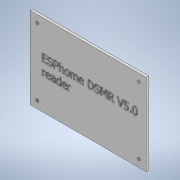
# Autodesk Inventor part: esp dsrm cover
Saved by Autodesk Inventor 2022.2 (Build 262287030, 287C)
## iProperties
Created: 2023-01-13
Part Number: esp dsrm cover
Material: Generic
Document SubType Name: Modeling
Designer: Ritchie
Density: 1 g/cm^3
Appearance: Default
Author: Ritchie
## iProperties of the stored document esp dsrm cover_3DPrint.ipt
Created: 2023-01-13
Part Number: esp dsrm cover_3DPrint
Material: Generic
Document SubType Name: Modeling
Designer: Ritchie
Density: 1 g/cm^3
Appearance: Default
Author: Ritchie
Autodesk Inventor part; units mm, degrees
ref_plane "YZ Plane" through (0, 0, 0) normal (1, 0, 0) x (0, 1, 0)
ref_plane "XZ Plane" through (0, 0, 0) normal (0, 1, 0) x (-1, 0, 0)
ref_plane "XY Plane" through (0, 0, 0) normal (0, 0, 1) x (1, 0, 0)
derived "esp_housing_dsrm.ipt"
sketch "Sketch15" plane through (0, 0, 33) normal (0, 0, 1) x (1, 0, 0)
  circle A0 centre (-9, 1) radius 1
  circle A1 centre (74.024, 55.742) radius 1
  circle A2 centre (-9, 55.742) radius 1
  arc A3 (77.024, 1) -> (74.024, -2) centre (74.024, 1) ccw
  line L0 (77.024, 1) -> (77.024, 55.742)
  arc A4 (74.024, 58.742) -> (77.024, 55.742) centre (74.024, 55.742) ccw
  line L1 (74.024, 58.742) -> (-9, 58.742)
  arc A5 (-12, 55.742) -> (-9, 58.742) centre (-9, 55.742) ccw
  line L2 (-12, 55.742) -> (-12, 1)
  arc A6 (-9, -2) -> (-12, 1) centre (-9, 1) ccw
  line L3 (-9, -2) -> (74.024, -2)
  circle A7 centre (74.024, 1) radius 1
  line L4 (-14, -4) -> (79.024, -4)
  line L5 (79.024, -4) -> (79.024, 60.742)
  line L6 (79.024, 60.742) -> (-14, 60.742)
  line L7 (-14, 60.742) -> (-14, -4)
  line L8 (-15, -5) -> (-15, 61.742)
  line L9 (-15, 61.742) -> (80.024, 61.742)
  line L10 (80.024, 61.742) -> (80.024, -5)
  line L11 (80.024, -5) -> (-15, -5)
  point P0 (0, 0)
extrude "Extrusion1" add sketch "Sketch15" along normal blind 2 contours A0 | A1 | A2 | A3 L3 A6 L2 A5 L1 A4 L0 | A7 | L7 L6 L5 L4 | L8 L9 L10 L11
extrude "Extrusion2" add sketch "Sketch15" against normal blind 1 contours A0 | A1 | A2 | A3 L3 A6 L2 A5 L1 A4 L0 | A7 | L7 L6 L5 L4
hole "Hole1" at (-9, 1, 33) at (74.024, 1, 33) at (74.024, 55.742, 33) at (-9, 55.742, 33) direction (0, 0, -1) diameter 2.4 end through all both
sketch "Sketch2" plane through (-15, 61.742, 35) normal (0, 0, 1) x (1, 0, 0)
  line L0 (9.4633, -24.8281) -> (88.4466, -24.8281) construction
  line L1 (88.4466, -24.8281) -> (88.4466, -45.4167) construction
  line L2 (88.4466, -45.4167) -> (9.4633, -45.4167) construction
  line L3 (9.4633, -45.4167) -> (9.4633, -24.8281) construction
  line L4 (10.0812, -31.1999) -> (10.0812, -25.0999)
  line L5 (10.0812, -25.0999) -> (13.8974, -25.0999)
  line L6 (13.8974, -25.0999) -> (13.8974, -25.8217)
  line L7 (13.8974, -25.8217) -> (10.8919, -25.8217)
  line L8 (10.8919, -25.8217) -> (10.8919, -27.4925)
  line L9 (10.8919, -27.4925) -> (13.6947, -27.4925)
  line L10 (13.6947, -27.4925) -> (13.6947, -28.2142)
  line L11 (13.6947, -28.2142) -> (10.8919, -28.2142)
  line L12 (10.8919, -28.2142) -> (10.8919, -30.4782)
  line L13 (10.8919, -30.4782) -> (13.8974, -30.4782)
  line L14 (13.8974, -30.4782) -> (13.8974, -31.1999)
  line L15 (13.8974, -31.1999) -> (10.0812, -31.1999)
  spline S0 degree 2 poles (16.4877, -31.3087) (15.8253, -31.3087) (14.8959, -31.0319) (14.4856, -30.8341) knots 0 0 0 1 2 2 2
  line L16 (14.4856, -30.8341) -> (14.4856, -29.8158)
  line L17 (14.4856, -29.8158) -> (14.545, -29.8158)
  spline S1 degree 2 poles (14.545, -29.8158) (14.9454, -30.1915) (15.9587, -30.6067) (16.4284, -30.6067) knots 0 0 0 1 2 2 2
  spline S2 degree 2 poles (16.4284, -30.6067) (17.1006, -30.6067) (17.7878, -30.0482) (17.7878, -29.5884) knots 0 0 0 1 2 2 2
  spline S3 degree 2 poles (17.7878, -29.5884) (17.7878, -29.2226) (17.4269, -28.7678) (17.0364, -28.6541) knots 0 0 0 1 2 2 2
  spline S4 degree 2 poles (17.0364, -28.6541) (16.7546, -28.5751) (16.285, -28.4663) (15.934, -28.3773) knots 0 0 0 1 2 2 2
  spline S5 degree 2 poles (15.934, -28.3773) (15.6177, -28.2933) (15.1184, -28.0412) (14.9256, -27.8385) knots 0 0 0 1 2 2 2
  spline S6 degree 2 poles (14.9256, -27.8385) (14.7378, -27.6358) (14.5301, -27.0921) (14.5301, -26.7362) knots 0 0 0 1 2 2 2
  spline S7 degree 2 poles (14.5301, -26.7362) (14.5301, -25.9947) (15.6869, -24.9912) (16.5816, -24.9912) knots 0 0 0 1 2 2 2
  spline S8 degree 2 poles (16.5816, -24.9912) (17.0957, -24.9912) (18.0053, -25.1939) (18.3958, -25.3866) knots 0 0 0 1 2 2 2
  line L18 (18.3958, -25.3866) -> (18.3958, -26.3555)
  line L19 (18.3958, -26.3555) -> (18.3365, -26.3555)
  spline S9 degree 2 poles (18.3365, -26.3555) (18.0448, -26.0886) (17.1352, -25.6931) (16.636, -25.6931) knots 0 0 0 1 2 2 2
  spline S10 degree 2 poles (16.636, -25.6931) (16.0724, -25.6931) (15.3754, -26.2221) (15.3754, -26.6521) knots 0 0 0 1 2 2 2
  spline S11 degree 2 poles (15.3754, -26.6521) (15.3754, -27.0377) (15.7857, -27.4974) (16.1713, -27.6012) knots 0 0 0 1 2 2 2
  spline S12 degree 2 poles (16.1713, -27.6012) (16.4284, -27.6704) (17.1748, -27.8484) (17.422, -27.9225) knots 0 0 0 1 2 2 2
  spline S13 degree 2 poles (17.422, -27.9225) (18.0497, -28.1153) (18.6331, -28.8914) (18.6331, -29.4599) knots 0 0 0 1 2 2 2
  spline S14 degree 2 poles (18.6331, -29.4599) (18.6331, -29.8208) (18.3414, -30.5128) (18.0794, -30.755) knots 0 0 0 1 2 2 2
  spline S15 degree 2 poles (18.0794, -30.755) (17.7878, -31.022) (17.0463, -31.3087) (16.4877, -31.3087) knots 0 0 0 1 2 2 2
  spline S16 degree 2 poles (23.3143, -26.9388) (23.3143, -27.3343) (23.0326, -28.0461) (22.7805, -28.2933) knots 0 0 0 1 2 2 2
  spline S17 degree 2 poles (22.7805, -28.2933) (22.4641, -28.6047) (21.6089, -28.926) (20.9564, -28.926) knots 0 0 0 1 2 2 2
  line L20 (20.9564, -28.926) -> (20.2693, -28.926)
  line L21 (20.2693, -28.926) -> (20.2693, -31.1999)
  line L22 (20.2693, -31.1999) -> (19.4586, -31.1999)
  line L23 (19.4586, -31.1999) -> (19.4586, -25.0999)
  line L24 (19.4586, -25.0999) -> (20.991, -25.0999)
  spline S18 degree 2 poles (20.991, -25.0999) (21.5348, -25.0999) (22.296, -25.2779) (22.5877, -25.4806) knots 0 0 0 1 2 2 2
  spline S19 degree 2 poles (22.5877, -25.4806) (22.9288, -25.7129) (23.3143, -26.4297) (23.3143, -26.9388) knots 0 0 0 1 2 2 2
  spline S20 degree 2 poles (22.469, -26.9635) (22.469, -26.6472) (22.2515, -26.1825) (22.0291, -26.0342) knots 0 0 0 1 2 2 2
  spline S21 degree 2 poles (22.0291, -26.0342) (21.8363, -25.9057) (21.3222, -25.8019) (20.9416, -25.8019) knots 0 0 0 1 2 2 2
  line L25 (20.9416, -25.8019) -> (20.2693, -25.8019)
  line L26 (20.2693, -25.8019) -> (20.2693, -28.234)
  line L27 (20.2693, -28.234) -> (20.8229, -28.234)
  spline S22 degree 2 poles (20.8229, -28.234) (21.3173, -28.234) (21.9253, -28.0758) (22.123, -27.8682) knots 0 0 0 1 2 2 2
  spline S23 degree 2 poles (22.123, -27.8682) (22.3059, -27.6853) (22.469, -27.2552) (22.469, -26.9635) knots 0 0 0 1 2 2 2
  line L28 (27.6199, -31.1999) -> (26.8488, -31.1999)
  line L29 (26.8488, -31.1999) -> (26.8488, -28.5899)
  spline S24 degree 2 poles (26.8488, -28.5899) (26.8488, -28.2735) (26.7895, -27.7298) (26.7005, -27.5666) knots 0 0 0 1 2 2 2
  spline S25 degree 2 poles (26.7005, -27.5666) (26.6066, -27.3936) (26.2704, -27.2255) (25.9837, -27.2255) knots 0 0 0 1 2 2 2
  spline S26 degree 2 poles (25.9837, -27.2255) (25.697, -27.2255) (25.089, -27.532) (24.7973, -27.7792) knots 0 0 0 1 2 2 2
  line L30 (24.7973, -27.7792) -> (24.7973, -31.1999)
  line L31 (24.7973, -31.1999) -> (24.0262, -31.1999)
  line L32 (24.0262, -31.1999) -> (24.0262, -24.8281)
  line L33 (24.0262, -24.8281) -> (24.7973, -24.8281)
  line L34 (24.7973, -24.8281) -> (24.7973, -27.1316)
  spline S27 degree 2 poles (24.7973, -27.1316) (25.1433, -26.8202) (25.8107, -26.4939) (26.1864, -26.4939) knots 0 0 0 1 2 2 2
  spline S28 degree 2 poles (26.1864, -26.4939) (26.8587, -26.4939) (27.6199, -27.3837) (27.6199, -28.229) knots 0 0 0 1 2 2 2
  line L35 (27.6199, -28.229) -> (27.6199, -31.1999)
  spline S29 degree 2 poles (32.4643, -28.9112) (32.4643, -30.0679) (31.3521, -31.3285) (30.4228, -31.3285) knots 0 0 0 1 2 2 2
  spline S30 degree 2 poles (30.4228, -31.3285) (29.4687, -31.3285) (28.3762, -30.0284) (28.3762, -28.9112) knots 0 0 0 1 2 2 2
  spline S31 degree 2 poles (28.3762, -28.9112) (28.3762, -27.7644) (29.5033, -26.4939) (30.4228, -26.4939) knots 0 0 0 1 2 2 2
  spline S32 degree 2 poles (30.4228, -26.4939) (31.3521, -26.4939) (32.4643, -27.7594) (32.4643, -28.9112) knots 0 0 0 1 2 2 2
  spline S33 degree 2 poles (31.6685, -28.9112) (31.6685, -28.0214) (31.0209, -27.1563) (30.4228, -27.1563) knots 0 0 0 1 2 2 2
  spline S34 degree 2 poles (30.4228, -27.1563) (29.8246, -27.1563) (29.1721, -28.0214) (29.1721, -28.9112) knots 0 0 0 1 2 2 2
  spline S35 degree 2 poles (29.1721, -28.9112) (29.1721, -29.7763) (29.8246, -30.6661) (30.4228, -30.6661) knots 0 0 0 1 2 2 2
  spline S36 degree 2 poles (30.4228, -30.6661) (31.016, -30.6661) (31.6685, -29.7911) (31.6685, -28.9112) knots 0 0 0 1 2 2 2
  line L36 (38.4457, -31.1999) -> (38.4457, -28.5503)
  spline S37 degree 2 poles (38.4457, -28.5503) (38.4457, -28.234) (38.3963, -27.6952) (38.3172, -27.5469) knots 0 0 0 1 2 2 2
  spline S38 degree 2 poles (38.3172, -27.5469) (38.2381, -27.3837) (37.9365, -27.2255) (37.6745, -27.2255) knots 0 0 0 1 2 2 2
  spline S39 degree 2 poles (37.6745, -27.2255) (37.4373, -27.2255) (36.8935, -27.5172) (36.6068, -27.794) knots 0 0 0 1 2 2 2
  spline S40 degree 2 poles (36.6068, -27.794) (36.6117, -27.8632) (36.6216, -28.056) (36.6216, -28.1845) knots 0 0 0 1 2 2 2
  line L37 (36.6216, -28.1845) -> (36.6216, -31.1999)
  line L38 (36.6216, -31.1999) -> (35.8505, -31.1999)
  line L39 (35.8505, -31.1999) -> (35.8505, -28.5503)
  spline S41 degree 2 poles (35.8505, -28.5503) (35.8505, -28.234) (35.801, -27.6952) (35.722, -27.5469) knots 0 0 0 1 2 2 2
  spline S42 degree 2 poles (35.722, -27.5469) (35.6429, -27.3837) (35.3413, -27.2255) (35.0793, -27.2255) knots 0 0 0 1 2 2 2
  spline S43 degree 2 poles (35.0793, -27.2255) (34.8322, -27.2255) (34.2835, -27.537) (34.0264, -27.7792) knots 0 0 0 1 2 2 2
  line L40 (34.0264, -27.7792) -> (34.0264, -31.1999)
  line L41 (34.0264, -31.1999) -> (33.2553, -31.1999)
  line L42 (33.2553, -31.1999) -> (33.2553, -26.6225)
  line L43 (33.2553, -26.6225) -> (34.0264, -26.6225)
  line L44 (34.0264, -26.6225) -> (34.0264, -27.1267)
  spline S44 degree 2 poles (34.0264, -27.1267) (34.3279, -26.8251) (34.9211, -26.4939) (35.2771, -26.4939) knots 0 0 0 1 2 2 2
  spline S45 degree 2 poles (35.2771, -26.4939) (35.6824, -26.4939) (36.3102, -26.8647) (36.4733, -27.2849) knots 0 0 0 1 2 2 2
  spline S46 degree 2 poles (36.4733, -27.2849) (36.8243, -26.8943) (37.4867, -26.4939) (37.8723, -26.4939) knots 0 0 0 1 2 2 2
  spline S47 degree 2 poles (37.8723, -26.4939) (38.1689, -26.4939) (38.6533, -26.6768) (38.8313, -26.8845) knots 0 0 0 1 2 2 2
  spline S48 degree 2 poles (38.8313, -26.8845) (39.0142, -27.0921) (39.2168, -27.7149) (39.2168, -28.1845) knots 0 0 0 1 2 2 2
  line L45 (39.2168, -28.1845) -> (39.2168, -31.1999)
  line L46 (39.2168, -31.1999) -> (38.4457, -31.1999)
  spline S49 degree 2 poles (42.2866, -31.3037) (41.1892, -31.3037) (39.9831, -30.0729) (39.9831, -28.9359) knots 0 0 0 1 2 2 2
  spline S50 degree 2 poles (39.9831, -28.9359) (39.9831, -27.8187) (41.1546, -26.4939) (42.0988, -26.4939) knots 0 0 0 1 2 2 2
  spline S51 degree 2 poles (42.0988, -26.4939) (42.5239, -26.4939) (43.1814, -26.7411) (43.4236, -27.0031) knots 0 0 0 1 2 2 2
  spline S52 degree 2 poles (43.4236, -27.0031) (43.6707, -27.2651) (43.9327, -28.0214) (43.9327, -28.5701) knots 0 0 0 1 2 2 2
  line L47 (43.9327, -28.5701) -> (43.9327, -28.9903)
  line L48 (43.9327, -28.9903) -> (40.7641, -28.9903)
  spline S53 degree 2 poles (40.7641, -28.9903) (40.7641, -29.7862) (41.5649, -30.6315) (42.2767, -30.6315) knots 0 0 0 1 2 2 2
  spline S54 degree 2 poles (42.2767, -30.6315) (42.5288, -30.6315) (43.0182, -30.5178) (43.216, -30.4288) knots 0 0 0 1 2 2 2
  spline S55 degree 2 poles (43.216, -30.4288) (43.4236, -30.3299) (43.7103, -30.1569) (43.8042, -30.0778) knots 0 0 0 1 2 2 2
  line L49 (43.8042, -30.0778) -> (43.8487, -30.0778)
  line L50 (43.8487, -30.0778) -> (43.8487, -30.9182)
  spline S56 degree 2 poles (43.8487, -30.9182) (43.7152, -30.9725) (43.3099, -31.1307) (43.1517, -31.1752) knots 0 0 0 1 2 2 2
  spline S57 degree 2 poles (43.1517, -31.1752) (42.9292, -31.2395) (42.5634, -31.3037) (42.2866, -31.3037) knots 0 0 0 1 2 2 2
  spline S58 degree 2 poles (43.1814, -28.402) (43.1715, -28.0906) (43.0429, -27.6358) (42.9194, -27.4826) knots 0 0 0 1 2 2 2
  spline S59 degree 2 poles (42.9194, -27.4826) (42.7859, -27.3096) (42.3657, -27.1267) (42.0543, -27.1267) knots 0 0 0 1 2 2 2
  spline S60 degree 2 poles (42.0543, -27.1267) (41.7478, -27.1267) (41.3177, -27.3096) (41.1398, -27.4875) knots 0 0 0 1 2 2 2
  spline S61 degree 2 poles (41.1398, -27.4875) (40.9668, -27.6704) (40.7888, -28.1104) (40.7641, -28.402) knots 0 0 0 1 2 2 2
  line L51 (40.7641, -28.402) -> (43.1814, -28.402)
  spline S62 degree 2 poles (52.2028, -28.1549) (52.2028, -28.9903) (51.5256, -30.3349) (50.9571, -30.7105) knots 0 0 0 1 2 2 2
  spline S63 degree 2 poles (50.9571, -30.7105) (50.4925, -31.0022) (49.5384, -31.1999) (48.7969, -31.1999) knots 0 0 0 1 2 2 2
  line L52 (48.7969, -31.1999) -> (47.393, -31.1999)
  line L53 (47.393, -31.1999) -> (47.393, -25.0999)
  line L54 (47.393, -25.0999) -> (48.7821, -25.0999)
  spline S64 degree 2 poles (48.7821, -25.0999) (49.6422, -25.0999) (50.621, -25.357) (50.967, -25.5844) knots 0 0 0 1 2 2 2
  spline S65 degree 2 poles (50.967, -25.5844) (51.5553, -25.9749) (52.2028, -27.2651) (52.2028, -28.1549) knots 0 0 0 1 2 2 2
  spline S66 degree 2 poles (51.3575, -28.145) (51.3575, -27.443) (50.8929, -26.4494) (50.4331, -26.1677) knots 0 0 0 1 2 2 2
  spline S67 degree 2 poles (50.4331, -26.1677) (50.1069, -25.9749) (49.3703, -25.8019) (48.8216, -25.8019) knots 0 0 0 1 2 2 2
  line L55 (48.8216, -25.8019) -> (48.2037, -25.8019)
  line L56 (48.2037, -25.8019) -> (48.2037, -30.498)
  line L57 (48.2037, -30.498) -> (48.8216, -30.498)
  spline S68 degree 2 poles (48.8216, -30.498) (49.3604, -30.498) (50.1761, -30.325) (50.5073, -30.0926) knots 0 0 0 1 2 2 2
  spline S69 degree 2 poles (50.5073, -30.0926) (50.9324, -29.8059) (51.3575, -28.8568) (51.3575, -28.145) knots 0 0 0 1 2 2 2
  spline S70 degree 2 poles (54.7832, -31.3087) (54.1208, -31.3087) (53.1915, -31.0319) (52.7812, -30.8341) knots 0 0 0 1 2 2 2
  line L58 (52.7812, -30.8341) -> (52.7812, -29.8158)
  line L59 (52.7812, -29.8158) -> (52.8405, -29.8158)
  spline S71 degree 2 poles (52.8405, -29.8158) (53.2409, -30.1915) (54.2543, -30.6067) (54.7239, -30.6067) knots 0 0 0 1 2 2 2
  spline S72 degree 2 poles (54.7239, -30.6067) (55.3962, -30.6067) (56.0833, -30.0482) (56.0833, -29.5884) knots 0 0 0 1 2 2 2
  spline S73 degree 2 poles (56.0833, -29.5884) (56.0833, -29.2226) (55.7224, -28.7678) (55.3319, -28.6541) knots 0 0 0 1 2 2 2
  spline S74 degree 2 poles (55.3319, -28.6541) (55.0502, -28.5751) (54.5805, -28.4663) (54.2296, -28.3773) knots 0 0 0 1 2 2 2
  spline S75 degree 2 poles (54.2296, -28.3773) (53.9132, -28.2933) (53.4139, -28.0412) (53.2211, -27.8385) knots 0 0 0 1 2 2 2
  spline S76 degree 2 poles (53.2211, -27.8385) (53.0333, -27.6358) (52.8257, -27.0921) (52.8257, -26.7362) knots 0 0 0 1 2 2 2
  spline S77 degree 2 poles (52.8257, -26.7362) (52.8257, -25.9947) (53.9824, -24.9912) (54.8771, -24.9912) knots 0 0 0 1 2 2 2
  spline S78 degree 2 poles (54.8771, -24.9912) (55.3912, -24.9912) (56.3008, -25.1939) (56.6913, -25.3866) knots 0 0 0 1 2 2 2
  line L60 (56.6913, -25.3866) -> (56.6913, -26.3555)
  line L61 (56.6913, -26.3555) -> (56.632, -26.3555)
  spline S79 degree 2 poles (56.632, -26.3555) (56.3403, -26.0886) (55.4308, -25.6931) (54.9315, -25.6931) knots 0 0 0 1 2 2 2
  spline S80 degree 2 poles (54.9315, -25.6931) (54.368, -25.6931) (53.671, -26.2221) (53.671, -26.6521) knots 0 0 0 1 2 2 2
  spline S81 degree 2 poles (53.671, -26.6521) (53.671, -27.0377) (54.0813, -27.4974) (54.4668, -27.6012) knots 0 0 0 1 2 2 2
  spline S82 degree 2 poles (54.4668, -27.6012) (54.7239, -27.6704) (55.4703, -27.8484) (55.7175, -27.9225) knots 0 0 0 1 2 2 2
  spline S83 degree 2 poles (55.7175, -27.9225) (56.3453, -28.1153) (56.9286, -28.8914) (56.9286, -29.4599) knots 0 0 0 1 2 2 2
  spline S84 degree 2 poles (56.9286, -29.4599) (56.9286, -29.8208) (56.6369, -30.5128) (56.375, -30.755) knots 0 0 0 1 2 2 2
  spline S85 degree 2 poles (56.375, -30.755) (56.0833, -31.022) (55.3418, -31.3087) (54.7832, -31.3087) knots 0 0 0 1 2 2 2
  line L62 (62.9841, -31.1999) -> (62.1734, -31.1999)
  line L63 (62.1734, -31.1999) -> (62.1734, -25.9452)
  line L64 (62.1734, -25.9452) -> (60.5817, -29.5192)
  line L65 (60.5817, -29.5192) -> (60.0873, -29.5192)
  line L66 (60.0873, -29.5192) -> (58.5104, -25.9452)
  line L67 (58.5104, -25.9452) -> (58.5104, -31.1999)
  line L68 (58.5104, -31.1999) -> (57.7541, -31.1999)
  line L69 (57.7541, -31.1999) -> (57.7541, -25.0999)
  line L70 (57.7541, -25.0999) -> (58.8614, -25.0999)
  line L71 (58.8614, -25.0999) -> (60.3839, -28.496)
  line L72 (60.3839, -28.496) -> (61.857, -25.0999)
  line L73 (61.857, -25.0999) -> (62.9841, -25.0999)
  line L74 (62.9841, -25.0999) -> (62.9841, -31.1999)
  line L75 (68.9408, -31.1999) -> (67.8878, -31.1999)
  line L76 (67.8878, -31.1999) -> (65.96, -28.7728)
  line L77 (65.96, -28.7728) -> (65.0306, -28.7728)
  line L78 (65.0306, -28.7728) -> (65.0306, -31.1999)
  line L79 (65.0306, -31.1999) -> (64.2199, -31.1999)
  line L80 (64.2199, -31.1999) -> (64.2199, -25.0999)
  line L81 (64.2199, -25.0999) -> (65.7919, -25.0999)
  spline S86 degree 2 poles (65.7919, -25.0999) (66.3159, -25.0999) (67.0228, -25.2136) (67.3441, -25.4212) knots 0 0 0 1 2 2 2
  spline S87 degree 2 poles (67.3441, -25.4212) (67.6654, -25.6289) (68.0361, -26.2764) (68.0361, -26.7559) knots 0 0 0 1 2 2 2
  spline S88 degree 2 poles (68.0361, -26.7559) (68.0361, -27.4233) (67.354, -28.3279) (66.7707, -28.5454) knots 0 0 0 1 2 2 2
  line L82 (66.7707, -28.5454) -> (68.9408, -31.1999)
  spline S89 degree 2 poles (67.1908, -26.8202) (67.1908, -26.5533) (67.003, -26.143) (66.8053, -26.0095) knots 0 0 0 1 2 2 2
  spline S90 degree 2 poles (66.8053, -26.0095) (66.6322, -25.8958) (66.1725, -25.8019) (65.8364, -25.8019) knots 0 0 0 1 2 2 2
  line L83 (65.8364, -25.8019) -> (65.0306, -25.8019)
  line L84 (65.0306, -25.8019) -> (65.0306, -28.0956)
  line L85 (65.0306, -28.0956) -> (65.7425, -28.0956)
  spline S91 degree 2 poles (65.7425, -28.0956) (66.0934, -28.0956) (66.652, -27.972) (66.8448, -27.7792) knots 0 0 0 1 2 2 2
  spline S92 degree 2 poles (66.8448, -27.7792) (67.0228, -27.6111) (67.1908, -27.1366) (67.1908, -26.8202) knots 0 0 0 1 2 2 2
  line L86 (76.4694, -25.0999) -> (74.3685, -31.1999)
  line L87 (74.3685, -31.1999) -> (73.4935, -31.1999)
  line L88 (73.4935, -31.1999) -> (71.3926, -25.0999)
  line L89 (71.3926, -25.0999) -> (72.2626, -25.0999)
  line L90 (72.2626, -25.0999) -> (73.9532, -30.1668)
  line L91 (73.9532, -30.1668) -> (75.6438, -25.0999)
  line L92 (75.6438, -25.0999) -> (76.4694, -25.0999)
  spline S93 degree 2 poles (80.5772, -29.2622) (80.5772, -29.7021) (80.2955, -30.4535) (80.0384, -30.7303) knots 0 0 0 1 2 2 2
  spline S94 degree 2 poles (80.0384, -30.7303) (79.7814, -31.0071) (79.0151, -31.3285) (78.5406, -31.3285) knots 0 0 0 1 2 2 2
  spline S95 degree 2 poles (78.5406, -31.3285) (78.1056, -31.3285) (77.2553, -31.1357) (76.9439, -30.9824) knots 0 0 0 1 2 2 2
  line L93 (76.9439, -30.9824) -> (76.9439, -30.1174)
  line L94 (76.9439, -30.1174) -> (77.0032, -30.1174)
  spline S96 degree 2 poles (77.0032, -30.1174) (77.0972, -30.1866) (77.4481, -30.3645) (77.6607, -30.4436) knots 0 0 0 1 2 2 2
  spline S97 degree 2 poles (77.6607, -30.4436) (77.9029, -30.5276) (78.3033, -30.6216) (78.5554, -30.6216) knots 0 0 0 1 2 2 2
  spline S98 degree 2 poles (78.5554, -30.6216) (78.8026, -30.6216) (79.2673, -30.4436) (79.4353, -30.2508) knots 0 0 0 1 2 2 2
  spline S99 degree 2 poles (79.4353, -30.2508) (79.5886, -30.0679) (79.7468, -29.5835) (79.7468, -29.2572) knots 0 0 0 1 2 2 2
  spline S100 degree 2 poles (79.7468, -29.2572) (79.7468, -28.931) (79.5688, -28.5157) (79.4007, -28.3773) knots 0 0 0 1 2 2 2
  spline S101 degree 2 poles (79.4007, -28.3773) (79.2277, -28.2241) (78.7136, -28.0956) (78.4022, -28.0956) knots 0 0 0 1 2 2 2
  spline S102 degree 2 poles (78.4022, -28.0956) (78.066, -28.0956) (77.3987, -28.1994) (77.196, -28.2439) knots 0 0 0 1 2 2 2
  line L95 (77.196, -28.2439) -> (77.196, -25.0999)
  line L96 (77.196, -25.0999) -> (80.5426, -25.0999)
  line L97 (80.5426, -25.0999) -> (80.5426, -25.8167)
  line L98 (80.5426, -25.8167) -> (77.982, -25.8167)
  line L99 (77.982, -25.8167) -> (77.982, -27.443)
  spline S103 degree 2 poles (77.982, -27.443) (78.1303, -27.4233) (78.417, -27.4084) (78.5356, -27.4084) knots 0 0 0 1 2 2 2
  spline S104 degree 2 poles (78.5356, -27.4084) (79.0053, -27.4084) (79.6528, -27.5617) (79.9494, -27.7891) knots 0 0 0 1 2 2 2
  spline S105 degree 2 poles (79.9494, -27.7891) (80.251, -28.0165) (80.5772, -28.7085) (80.5772, -29.2622) knots 0 0 0 1 2 2 2
  line L100 (82.7671, -31.1999) -> (81.7883, -31.1999)
  line L101 (81.7883, -31.1999) -> (81.7883, -30.0333)
  line L102 (81.7883, -30.0333) -> (82.7671, -30.0333)
  line L103 (82.7671, -30.0333) -> (82.7671, -31.1999)
  spline S106 degree 2 poles (87.7944, -28.1499) (87.7944, -29.7911) (86.8403, -31.3285) (85.8468, -31.3285) knots 0 0 0 1 2 2 2
  spline S107 degree 2 poles (85.8468, -31.3285) (84.8383, -31.3285) (83.8942, -29.7614) (83.8942, -28.1549) knots 0 0 0 1 2 2 2
  spline S108 degree 2 poles (83.8942, -28.1549) (83.8942, -26.5038) (84.8482, -24.9764) (85.8468, -24.9764) knots 0 0 0 1 2 2 2
  spline S109 degree 2 poles (85.8468, -24.9764) (86.8502, -24.9764) (87.7944, -26.5582) (87.7944, -28.1499) knots 0 0 0 1 2 2 2
  spline S110 degree 2 poles (86.7464, -30.0086) (86.8651, -29.7071) (86.9639, -28.7777) (86.9639, -28.1499) knots 0 0 0 1 2 2 2
  spline S111 degree 2 poles (86.9639, -28.1499) (86.9639, -27.5221) (86.8651, -26.5977) (86.7415, -26.2863) knots 0 0 0 1 2 2 2
  spline S112 degree 2 poles (86.7415, -26.2863) (86.6179, -25.9749) (86.1878, -25.6536) (85.8468, -25.6536) knots 0 0 0 1 2 2 2
  spline S113 degree 2 poles (85.8468, -25.6536) (85.5057, -25.6536) (85.0657, -25.9749) (84.9372, -26.2962) knots 0 0 0 1 2 2 2
  spline S114 degree 2 poles (84.9372, -26.2962) (84.8136, -26.6076) (84.7246, -27.5567) (84.7246, -28.1549) knots 0 0 0 1 2 2 2
  spline S115 degree 2 poles (84.7246, -28.1549) (84.7246, -28.7975) (84.8037, -29.6576) (84.9322, -29.9938) knots 0 0 0 1 2 2 2
  spline S116 degree 2 poles (84.9322, -29.9938) (85.0509, -30.3101) (85.4908, -30.6512) (85.8468, -30.6512) knots 0 0 0 1 2 2 2
  spline S117 degree 2 poles (85.8468, -30.6512) (86.1829, -30.6512) (86.6228, -30.3299) (86.7464, -30.0086) knots 0 0 0 1 2 2 2
  line L104 (12.449, -37.4915) -> (12.4095, -37.4915)
  spline S118 degree 2 poles (12.4095, -37.4915) (12.3205, -37.4668) (12.1277, -37.4569) (11.9942, -37.4569) knots 0 0 0 1 2 2 2
  spline S119 degree 2 poles (11.9942, -37.4569) (11.6828, -37.4569) (11.0698, -37.7288) (10.793, -37.9957) knots 0 0 0 1 2 2 2
  line L105 (10.793, -37.9957) -> (10.793, -41.2434)
  line L106 (10.793, -41.2434) -> (10.0219, -41.2434)
  line L107 (10.0219, -41.2434) -> (10.0219, -36.666)
  line L108 (10.0219, -36.666) -> (10.793, -36.666)
  line L109 (10.793, -36.666) -> (10.793, -37.3481)
  spline S120 degree 2 poles (10.793, -37.3481) (11.2132, -36.9724) (11.841, -36.666) (12.1376, -36.666) knots 0 0 0 1 2 2 2
  spline S121 degree 2 poles (12.1376, -36.666) (12.2562, -36.666) (12.3749, -36.6758) (12.449, -36.6907) knots 0 0 0 1 2 2 2
  line L110 (12.449, -36.6907) -> (12.449, -37.4915)
  spline S122 degree 2 poles (15.0344, -41.3472) (13.9369, -41.3472) (12.7308, -40.1164) (12.7308, -38.9794) knots 0 0 0 1 2 2 2
  spline S123 degree 2 poles (12.7308, -38.9794) (12.7308, -37.8622) (13.9023, -36.5374) (14.8465, -36.5374) knots 0 0 0 1 2 2 2
  spline S124 degree 2 poles (14.8465, -36.5374) (15.2716, -36.5374) (15.9291, -36.7846) (16.1713, -37.0466) knots 0 0 0 1 2 2 2
  spline S125 degree 2 poles (16.1713, -37.0466) (16.4185, -37.3086) (16.6805, -38.0649) (16.6805, -38.6136) knots 0 0 0 1 2 2 2
  line L111 (16.6805, -38.6136) -> (16.6805, -39.0338)
  line L112 (16.6805, -39.0338) -> (13.5118, -39.0338)
  spline S126 degree 2 poles (13.5118, -39.0338) (13.5118, -39.8296) (14.3126, -40.6749) (15.0245, -40.6749) knots 0 0 0 1 2 2 2
  spline S127 degree 2 poles (15.0245, -40.6749) (15.2766, -40.6749) (15.766, -40.5613) (15.9637, -40.4723) knots 0 0 0 1 2 2 2
  spline S128 degree 2 poles (15.9637, -40.4723) (16.1713, -40.3734) (16.458, -40.2004) (16.5519, -40.1213) knots 0 0 0 1 2 2 2
  line L113 (16.5519, -40.1213) -> (16.5964, -40.1213)
  line L114 (16.5964, -40.1213) -> (16.5964, -40.9617)
  spline S129 degree 2 poles (16.5964, -40.9617) (16.463, -41.016) (16.0576, -41.1742) (15.8994, -41.2187) knots 0 0 0 1 2 2 2
  spline S130 degree 2 poles (15.8994, -41.2187) (15.677, -41.283) (15.3112, -41.3472) (15.0344, -41.3472) knots 0 0 0 1 2 2 2
  spline S131 degree 2 poles (15.9291, -38.4455) (15.9192, -38.1341) (15.7907, -37.6793) (15.6671, -37.5261) knots 0 0 0 1 2 2 2
  spline S132 degree 2 poles (15.6671, -37.5261) (15.5336, -37.3531) (15.1134, -37.1702) (14.802, -37.1702) knots 0 0 0 1 2 2 2
  spline S133 degree 2 poles (14.802, -37.1702) (14.4955, -37.1702) (14.0655, -37.3531) (13.8875, -37.531) knots 0 0 0 1 2 2 2
  spline S134 degree 2 poles (13.8875, -37.531) (13.7145, -37.7139) (13.5365, -38.1539) (13.5118, -38.4455) knots 0 0 0 1 2 2 2
  line L115 (13.5118, -38.4455) -> (15.9291, -38.4455)
  spline S135 degree 2 poles (20.0122, -40.759) (19.9183, -40.8282) (19.6019, -41.0754) (19.4536, -41.1495) knots 0 0 0 1 2 2 2
  spline S136 degree 2 poles (19.4536, -41.1495) (19.251, -41.2583) (18.8703, -41.3719) (18.5243, -41.3719) knots 0 0 0 1 2 2 2
  spline S137 degree 2 poles (18.5243, -41.3719) (18.2425, -41.3719) (17.7334, -41.1594) (17.5406, -40.9666) knots 0 0 0 1 2 2 2
  spline S138 degree 2 poles (17.5406, -40.9666) (17.3577, -40.7788) (17.1352, -40.2251) (17.1352, -39.9186) knots 0 0 0 1 2 2 2
  spline S139 degree 2 poles (17.1352, -39.9186) (17.1352, -39.4441) (17.5356, -38.7718) (17.9707, -38.579) knots 0 0 0 1 2 2 2
  spline S140 degree 2 poles (17.9707, -38.579) (18.3562, -38.401) (19.4042, -38.2676) (20.0122, -38.233) knots 0 0 0 1 2 2 2
  line L116 (20.0122, -38.233) -> (20.0122, -38.0847)
  spline S141 degree 2 poles (20.0122, -38.0847) (20.0122, -37.8177) (19.8491, -37.4865) (19.7008, -37.3926) knots 0 0 0 1 2 2 2
  spline S142 degree 2 poles (19.7008, -37.3926) (19.5525, -37.2987) (19.1274, -37.2394) (18.9, -37.2394) knots 0 0 0 1 2 2 2
  spline S143 degree 2 poles (18.9, -37.2394) (18.6331, -37.2394) (17.9113, -37.3976) (17.5505, -37.5508) knots 0 0 0 1 2 2 2
  line L117 (17.5505, -37.5508) -> (17.506, -37.5508)
  line L118 (17.506, -37.5508) -> (17.506, -36.7648)
  spline S144 degree 2 poles (17.506, -36.7648) (17.7185, -36.7055) (18.5144, -36.5572) (18.9049, -36.5572) knots 0 0 0 1 2 2 2
  spline S145 degree 2 poles (18.9049, -36.5572) (19.3795, -36.5572) (20.0271, -36.7055) (20.2841, -36.8983) knots 0 0 0 1 2 2 2
  spline S146 degree 2 poles (20.2841, -36.8983) (20.5362, -37.0861) (20.7834, -37.6843) (20.7834, -38.1143) knots 0 0 0 1 2 2 2
  line L119 (20.7834, -38.1143) -> (20.7834, -41.2434)
  line L120 (20.7834, -41.2434) -> (20.0122, -41.2434)
  line L121 (20.0122, -41.2434) -> (20.0122, -40.759)
  line L122 (20.0122, -40.1164) -> (20.0122, -38.8459)
  spline S147 degree 2 poles (20.0122, -38.8459) (19.7354, -38.8707) (18.9, -38.9547) (18.638, -39.0338) knots 0 0 0 1 2 2 2
  spline S148 degree 2 poles (18.638, -39.0338) (18.3315, -39.1277) (17.9311, -39.5182) (17.9311, -39.8642) knots 0 0 0 1 2 2 2
  spline S149 degree 2 poles (17.9311, -39.8642) (17.9311, -40.2597) (18.376, -40.6601) (18.8011, -40.6601) knots 0 0 0 1 2 2 2
  spline S150 degree 2 poles (18.8011, -40.6601) (19.162, -40.6601) (19.7552, -40.3487) (20.0122, -40.1164) knots 0 0 0 1 2 2 2
  line L123 (25.3856, -41.2434) -> (24.6144, -41.2434)
  line L124 (24.6144, -41.2434) -> (24.6144, -40.7788)
  spline S151 degree 2 poles (24.6144, -40.7788) (24.4365, -40.9271) (24.1745, -41.1248) (23.9965, -41.2088) knots 0 0 0 1 2 2 2
  spline S152 degree 2 poles (23.9965, -41.2088) (23.8334, -41.2879) (23.4824, -41.3719) (23.2501, -41.3719) knots 0 0 0 1 2 2 2
  spline S153 degree 2 poles (23.2501, -41.3719) (22.8744, -41.3719) (22.2416, -41.0605) (22.0192, -40.759) knots 0 0 0 1 2 2 2
  spline S154 degree 2 poles (22.0192, -40.759) (21.7967, -40.4574) (21.5496, -39.5677) (21.5496, -38.9893) knots 0 0 0 1 2 2 2
  spline S155 degree 2 poles (21.5496, -38.9893) (21.5496, -38.3862) (21.861, -37.5063) (22.1329, -37.1751) knots 0 0 0 1 2 2 2
  spline S156 degree 2 poles (22.1329, -37.1751) (22.385, -36.8785) (23.0919, -36.5374) (23.4824, -36.5374) knots 0 0 0 1 2 2 2
  spline S157 degree 2 poles (23.4824, -36.5374) (23.8235, -36.5374) (24.3326, -36.6907) (24.6144, -36.8489) knots 0 0 0 1 2 2 2
  line L125 (24.6144, -36.8489) -> (24.6144, -34.8715)
  line L126 (24.6144, -34.8715) -> (25.3856, -34.8715)
  line L127 (25.3856, -34.8715) -> (25.3856, -41.2434)
  line L128 (24.6144, -40.1312) -> (24.6144, -37.4865)
  spline S158 degree 2 poles (24.6144, -37.4865) (24.3277, -37.3481) (23.8729, -37.2443) (23.6109, -37.2443) knots 0 0 0 1 2 2 2
  spline S159 degree 2 poles (23.6109, -37.2443) (23.0177, -37.2443) (22.3455, -38.1341) (22.3455, -38.9745) knots 0 0 0 1 2 2 2
  spline S160 degree 2 poles (22.3455, -38.9745) (22.3455, -39.7852) (22.8596, -40.6403) (23.428, -40.6403) knots 0 0 0 1 2 2 2
  spline S161 degree 2 poles (23.428, -40.6403) (23.7296, -40.6403) (24.3425, -40.3635) (24.6144, -40.1312) knots 0 0 0 1 2 2 2
  spline S162 degree 2 poles (28.4899, -41.3472) (27.3925, -41.3472) (26.1864, -40.1164) (26.1864, -38.9794) knots 0 0 0 1 2 2 2
  spline S163 degree 2 poles (26.1864, -38.9794) (26.1864, -37.8622) (27.3579, -36.5374) (28.3021, -36.5374) knots 0 0 0 1 2 2 2
  spline S164 degree 2 poles (28.3021, -36.5374) (28.7272, -36.5374) (29.3847, -36.7846) (29.6269, -37.0466) knots 0 0 0 1 2 2 2
  spline S165 degree 2 poles (29.6269, -37.0466) (29.8741, -37.3086) (30.1361, -38.0649) (30.1361, -38.6136) knots 0 0 0 1 2 2 2
  line L129 (30.1361, -38.6136) -> (30.1361, -39.0338)
  line L130 (30.1361, -39.0338) -> (26.9674, -39.0338)
  spline S166 degree 2 poles (26.9674, -39.0338) (26.9674, -39.8296) (27.7682, -40.6749) (28.4801, -40.6749) knots 0 0 0 1 2 2 2
  spline S167 degree 2 poles (28.4801, -40.6749) (28.7322, -40.6749) (29.2215, -40.5613) (29.4193, -40.4723) knots 0 0 0 1 2 2 2
  spline S168 degree 2 poles (29.4193, -40.4723) (29.6269, -40.3734) (29.9136, -40.2004) (30.0075, -40.1213) knots 0 0 0 1 2 2 2
  line L131 (30.0075, -40.1213) -> (30.052, -40.1213)
  line L132 (30.052, -40.1213) -> (30.052, -40.9617)
  spline S169 degree 2 poles (30.052, -40.9617) (29.9185, -41.016) (29.5132, -41.1742) (29.355, -41.2187) knots 0 0 0 1 2 2 2
  spline S170 degree 2 poles (29.355, -41.2187) (29.1326, -41.283) (28.7668, -41.3472) (28.4899, -41.3472) knots 0 0 0 1 2 2 2
  spline S171 degree 2 poles (29.3847, -38.4455) (29.3748, -38.1341) (29.2463, -37.6793) (29.1227, -37.5261) knots 0 0 0 1 2 2 2
  spline S172 degree 2 poles (29.1227, -37.5261) (28.9892, -37.3531) (28.569, -37.1702) (28.2576, -37.1702) knots 0 0 0 1 2 2 2
  spline S173 degree 2 poles (28.2576, -37.1702) (27.9511, -37.1702) (27.5211, -37.3531) (27.3431, -37.531) knots 0 0 0 1 2 2 2
  spline S174 degree 2 poles (27.3431, -37.531) (27.1701, -37.7139) (26.9921, -38.1539) (26.9674, -38.4455) knots 0 0 0 1 2 2 2
  line L133 (26.9674, -38.4455) -> (29.3847, -38.4455)
  line L134 (33.3442, -37.4915) -> (33.3047, -37.4915)
  spline S175 degree 2 poles (33.3047, -37.4915) (33.2157, -37.4668) (33.0229, -37.4569) (32.8895, -37.4569) knots 0 0 0 1 2 2 2
  spline S176 degree 2 poles (32.8895, -37.4569) (32.578, -37.4569) (31.9651, -37.7288) (31.6882, -37.9957) knots 0 0 0 1 2 2 2
  line L135 (31.6882, -37.9957) -> (31.6882, -41.2434)
  line L136 (31.6882, -41.2434) -> (30.9171, -41.2434)
  line L137 (30.9171, -41.2434) -> (30.9171, -36.666)
  line L138 (30.9171, -36.666) -> (31.6882, -36.666)
  line L139 (31.6882, -36.666) -> (31.6882, -37.3481)
  spline S177 degree 2 poles (31.6882, -37.3481) (32.1084, -36.9724) (32.7362, -36.666) (33.0328, -36.666) knots 0 0 0 1 2 2 2
  spline S178 degree 2 poles (33.0328, -36.666) (33.1514, -36.666) (33.2701, -36.6758) (33.3442, -36.6907) knots 0 0 0 1 2 2 2
  line L140 (33.3442, -36.6907) -> (33.3442, -37.4915)
  point P0 (15, -61.742)
  constraints: 2 other
extrude "Extrusion3" cut sketch "Sketch2" against normal blind 1
body "Solid1"
